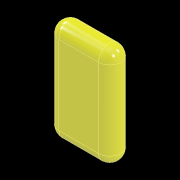
# Autodesk Inventor part: 模擬商品
Saved by Autodesk Inventor 2020 (Build 240168000, 168)
## iProperties
Created: 2021-04-13
Part Number: 模擬商品
Material: 一般
Document SubType Name: Modeling
Designer: 88690
Density: 1 g/cm^3
Appearance: 黃
Author: 88690
Autodesk Inventor part; units mm, degrees
ref_plane "XZ Plane" through (0, 0, 0) normal (0, 1, 0) x (-1, 0, 0)
ref_plane "XY Plane" through (0, 0, 0) normal (0, 0, 1) x (1, 0, 0)
sketch "草圖1" plane through (0, 0, 0) normal (0, 0, 1) x (1, 0, 0)
  line L0 (-55, 115) -> (55, 115)
  line L1 (55, 115) -> (55, -65)
  line L2 (55, -65) -> (-55, -65)
  line L3 (-55, -65) -> (-55, 115)
  line L4 (-55, 115) -> (55, -65) construction
  line L5 (55, 115) -> (-55, -65) construction
  line L6 (0, 0) -> (0, -31.0112) construction
  line L7 (0, 151) -> (0, -101) projected
  point P0 (0, 25)
  point P1 (0, 25)
  dimension "d0" = 110
  dimension "d1" = 180
  dimension "d7" = 25
  constraints: 14 end point, 4 midpoint, 2 parallel, 1 horizontal, 1 perpendicular, 1 vertical
  measures "d0" distance of L1.end L2.end
  measures "d1" distance of L0.end L1.end
  measures "d7" distance of L6.start point (0, 25)
extrude "擠出1" add sketch "草圖1" along normal mid plane 40
fillet "圓角1" radius 20 4 edges at (55, 115, 0) (-55, 115, 0) (55, -65, 0) (-55, -65, 0)
fillet "圓角2" radius 20 16 edges at (49.1421, 109.1421, 20) (0, 115, 20) (-49.1421, 109.1421, 20) (-55, 25, 20) (-49.1421, -59.1421, 20) (0, -65, 20) (49.1421, -59.1421, 20) (55, 25, 20) (0, 115, -20) (-49.1421, 109.1421, -20) (-55, 25, -20) (-49.1421, -59.1421, -20) (0, -65, -20) (49.1421, -59.1421, -20) (55, 25, -20) (49.1421, 109.1421, -20)
ref_plane "工作平面1" through (-12, 0, 0) normal (1, 0, 0) x (0, 1, 0)
